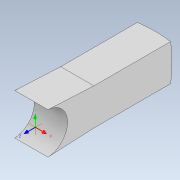
# Autodesk Inventor part: shank_inventor
Saved by Autodesk Inventor 2020 (Build 240168000, 168)
## iProperties
Created: 2021-01-07
Part Number: shank_inventor
Material: Generic
Document SubType Name: Modeling
Designer: DELL
Density: 1 g/cm^3
Appearance: Default
Author: DELL
Autodesk Inventor part; units mm, degrees
ref_plane "YZ Plane" through (0, 0, 0) normal (1, 0, 0) x (0, 1, 0)
ref_plane "XY Plane" through (0, 0, 0) normal (0, 0, 1) x (1, 0, 0)
ref_plane "UCS1: YZ Plane" through (0, 0, 0) normal (1, 0, 0) x (0, 1, 0)
sketch "Sketch2" plane through (0, 0, 0) normal (1, 0, 0) x (0, 1, 0)
  circle A0 centre (0, -70) radius 27.5
  line L0 (27.5, -190) -> (-27.5, -190)
  line L1 (0, -70) -> (0, -190) construction
  line L2 (-27.5, -70) -> (-27.5, -190)
  line L3 (27.5, -70) -> (27.5, -190)
  circle A1 centre (0, 0) radius 31
  line L4 (-30.9612, -1.55) -> (-27.4656, -71.375)
  line L5 (30.9612, -1.55) -> (27.4656, -71.375)
  line L6 (31.0388, 0) -> (-31.0388, 0)
  point P0 (-31, 0)
  point P1 (31, 0)
  point P2 (-31, 0)
  point P3 (-27.5, -70.6879)
  point P4 (27.5, -70.6879)
  dimension "d1" = 55
  dimension "d3" = 55
  dimension "d25" = 120
  dimension "d26" = 62
  dimension "d33" = 70
  constraints: 14 end point, 7 point on circle, 5 tangent, 2 centre point, 2 horizontal, 2 midpoint, 2 point on line, 1 coincident, 1 perpendicular, 1 vertical alignment, 1 other
  measures "d1" diameter of A0
  measures "d3" distance of L0.start L0.end
  measures "d25" distance from line of L0 L1.start
  measures "d26" diameter of A1
  measures "d33" distance of L1.start A1.centre
extrude "Extrusion1" add sketch "Sketch2" along normal blind 17.5 and the other way blind 32.5 contours A0
extrude "Extrusion2" add sketch "Sketch2" against normal blind 50 from surface at 17.5 contours L3 L5 A0 | A0 L4 L2 | L5 L3 L0 L2 L4 A0
sketch "Sketch5" plane through (17.5, -27.5, -190) normal (0, 0, -1) x (-1, 0, 0)
  circle A0 centre (25, 27.5) radius 10
  line L0 (50, 55) -> (50, 0) projected
  line L1 (0, 55) -> (50, 55) projected
  point P0 (17.5, 27.5)
  point P1 (50, 27.5)
  point P2 (-45, 0)
  point P3 (25, 55)
  dimension "d22" = 20
  constraints: 1 centre point, 1 horizontal alignment, 1 midpoint, 1 vertical alignment, 2 other
  measures "d22" diameter of A0
extrude "Extrusion4" cut sketch "Sketch5" against normal blind 60
ref_plane "Work Plane1" through (-7.5, 0, -70) normal (-1, 0, 0) x (0, 0, -1)
sketch "Sketch4" plane through (-7.5, 0, -70) normal (-1, 0, 0) x (0, 0, -1)
  circle A0 centre (-70, 0) radius 190
  line L0 (120, -27.5) -> (120, 27.5) projected
  line L1 (-260, 0) -> (120, 0)
  line L2 (120, 0) -> (120, 27.5)
  line L3 (120, 27.5) -> (0, 27.5) projected
  line L4 (120, 27.5) -> (120, 47.2424)
  line L5 (120, 47.2424) -> (114.033, 47.2424)
  point P0 (-70, 0)
  point P1 (117.9993, 27.5)
  point P2 (120, 0)
  constraints: 8 end point, 2 midpoint, 2 perpendicular, 2 point on circle, 1 centre point, 1 coincident, 1 tangent, 1 vertical
revolve "Revolution1" cut sketch "Sketch4" angle 360 about axis through (-7.5, 0, 190) along (0, 0, -1) contours L5 L4 L3 A0 | L3 L0 A0
extrude "Extrusion5" add sketch "Sketch2" along normal blind 17.5 and the other way blind 32.5 contours A0 L2 L4 A1 L5 L3
body "Solid1"
